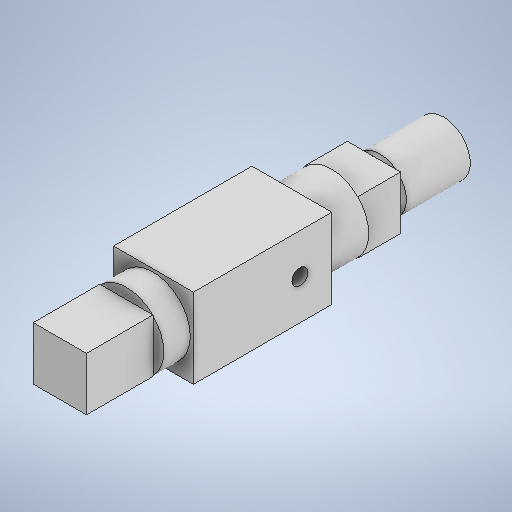
# Autodesk Inventor part: Pieza 9
Saved by Autodesk Inventor 2025.3 (Build 293356030, 356C)
## iProperties
Created: 2025-08-24
Part Number: Pieza 9
Material: Generic
Document SubType Name: Modeling
Designer: PC
Density: 1 g/cm^3
Appearance: Default
Author: PC
Autodesk Inventor part; units mm, degrees
ref_plane "YZ Plane" through (0, 0, 0) normal (1, 0, 0) x (0, 1, 0)
ref_plane "XZ Plane" through (0, 0, 0) normal (0, 1, 0) x (-1, 0, 0)
sketch "Sketch1" plane through (0, 0, 0) normal (0, 0, 1) x (1, 0, 0)
  line L0 (0, 0) -> (-15, 0)
  line L1 (-15, 0) -> (-15, 15)
  line L2 (-15, 15) -> (0, 15)
  line L3 (0, 15) -> (0, 0)
  dimension "d0" = 15
  dimension "d1" = 15
  constraints: 8 end point, 2 parallel, 1 horizontal, 1 perpendicular
  measures "d0" distance of L1.end L2.end
  measures "d1" distance of L0.end L1.end
extrude "Extrusion1" add sketch "Sketch1" along normal blind 26
sketch "Sketch2" plane through (0, 0, 26) normal (0, 0, 1) x (1, 0, 0)
  circle A0 centre (-7.5819, 7.5) radius 7
  point P0 (0, 0)
  dimension "d4" = 14
  constraints: 1 centre point, 1 coincident
  measures "d4" diameter of A0
extrude "Extrusion2" add sketch "Sketch2" along normal blind 5
sketch "Sketch3" plane through (-7.5819, 7.5, 31) normal (0, 0, 1) x (1, 0, 0)
  line L0 (-5, 5) -> (5, 5)
  line L1 (5, 5) -> (5, -5)
  line L2 (5, -5) -> (-5, -5)
  line L3 (-5, -5) -> (-5, 5)
  line L4 (-5, 5) -> (5, -5) construction
  line L5 (5, 5) -> (-5, -5) construction
  point P0 (7.5819, -7.5)
  point P1 (0, 0)
  dimension "d7" = 10
  dimension "d8" = 10
  constraints: 12 end point, 2 midpoint, 2 parallel, 1 horizontal, 1 perpendicular
  measures "d7" distance of L1.end L2.end
  measures "d8" distance of L0.end L1.end
extrude "Extrusion3" add sketch "Sketch3" along normal blind 12.5
sketch "Sketch4" plane through (0, 0, 0) normal (0, 0, -1) x (-1, 0, 0)
  circle A0 centre (7.5819, 7.5) radius 7 projected
  circle A1 centre (7.5819, 7.5) radius 7
  point P0 (0, 0)
  dimension "d11" = 14
  constraints: 2 coincident, 1 centre point
  measures "d11" diameter of A1
extrude "Extrusion4" add sketch "Sketch4" along normal blind 7.5
sketch "Sketch5" plane through (-7.5819, 7.5, -7.5) normal (0, 0, -1) x (-1, 0, 0)
  line L0 (-5, -5) -> (5, -5)
  line L1 (5, -5) -> (5, 5)
  line L2 (5, 5) -> (-5, 5)
  line L3 (-5, 5) -> (-5, -5)
  line L4 (-5, -5) -> (5, 5) construction
  line L5 (5, -5) -> (-5, 5) construction
  point P0 (-7.5819, -7.5)
  point P1 (0, 0)
  dimension "d14" = 10
  dimension "d15" = 10
  constraints: 12 end point, 2 midpoint, 2 parallel, 1 horizontal, 1 perpendicular
  measures "d14" distance of L2.end L1.end
  measures "d15" distance of L1.end L0.end
extrude "Extrusion5" add sketch "Sketch5" along normal blind 8
ref_plane "Work Plane1" through (-7.5, 0, 0) normal (-1, 0, 0) x (0, 0, 1)
sketch "Sketch6" plane through (-7.5, 0, 0) normal (-1, 0, 0) x (0, 0, 1)
  line L0 (-15.5, 12.5) -> (-15.5, 2.5) projected
  line L1 (-7.5, 2.5) -> (-15.5, 2.5) projected
  arc A0 (-15.5, 2.5) -> (-16.5, 2.5) centre (-16, 2.5) ccw
  line L2 (-28.5, 2.5) -> (-16.5, 2.5)
  arc A1 (-30.0167, 7.5) -> (-28.5, 2.5) centre (-21.0167, 7.5) ccw
  line L3 (-30.0167, 7.5) -> (-15.5, 7.5)
  line L4 (-15.5, 2.5) -> (-15.5, 7.5)
  point P0 (0, 0)
  dimension "d19" = 0.5
  dimension "d20" = 1
  dimension "d21" = 12
  dimension "d22" = 18
  constraints: 6 end point, 4 point on circle, 2 centre point, 1 coincident, 1 collinear, 1 horizontal, 1 midpoint, 1 tangent
  measures "d19" distance of L0.end point (-16, 2.5)
  measures "d20" diameter of A0
  measures "d21" distance of L2.start L2.end
  measures "d22" diameter of A1
revolve "Revolution1" add sketch "Sketch6" angle 360 about axis through (-7.5, 7.5, -30.0167) along (0, 0, 1)
sketch "Sketch7" plane through (-15, 0, 0) normal (-1, 0, 0) x (0, 0, 1)
  line L0 (0, 15) -> (26, 15) projected
  line L1 (0, 15) -> (0, 0) projected
  point P0 (6, 7.5)
  dimension "d31" = 7.5
  dimension "d32" = 6
  measures "d31" distance from line of L0 point (6, 7.5)
  measures "d32" distance from line of point (6, 7.5) L1
hole "Hole1" at (-15, 7.5, 6) direction (1, 0, 0) diameter 3 end through all
body "Solid1"
